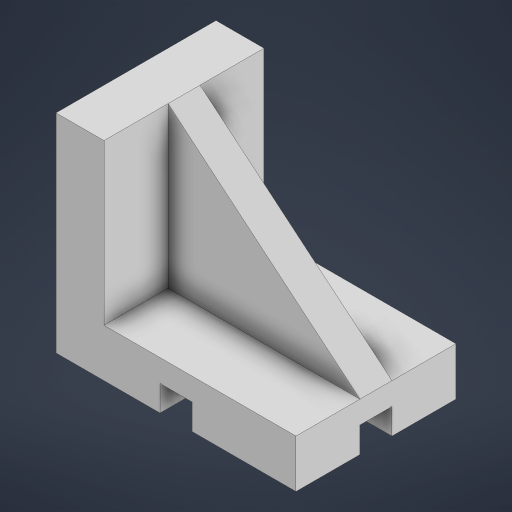
# Autodesk Inventor part: Part2
Saved by Autodesk Inventor 2023 (Build 270158000, 158)
## iProperties
Created: 2023-04-25
Part Number: Part2
Material: Ogólny
Document SubType Name: Modeling
Designer: Adam
Density: 1 g/cm^3
Appearance: Domyślna
Author: Adam
Autodesk Inventor part; units mm, degrees
ref_plane "YZ Plane" through (0, 0, 0) normal (1, 0, 0) x (0, 1, 0)
ref_plane "XZ Plane" through (0, 0, 0) normal (0, 1, 0) x (-1, 0, 0)
ref_plane "XY Plane" through (0, 0, 0) normal (0, 0, 1) x (1, 0, 0)
sketch "Szkic6" plane through (0, 0, 0) normal (0, 0, 1) x (1, 0, 0)
  point P0 (0, 0)
sketch "Szkic7" plane through (0, 0, 0) normal (0, 0, 1) x (1, 0, 0)
  line L0 (0, 65) -> (0, 0)
  line L1 (0, 0) -> (75, 0)
  line L2 (75, 0) -> (75, 15)
  line L3 (75, 15) -> (15, 15)
  line L4 (15, 15) -> (15, 65)
  line L5 (15, 65) -> (0, 65)
  dimension "d13" = 65
  dimension "d14" = 75
  dimension "d15" = 15
  dimension "d16" = 15
  constraints: 12 end point, 5 perpendicular, 1 vertical
  measures "d13" distance of L0.start L0.end
  measures "d14" distance of L0.end L1.end
  measures "d15" distance of L1.end L2.end
  measures "d16" distance of L4.end L0.start
extrude "Wyciągnięcie proste3" add sketch "Szkic7" along normal mid plane 50
sketch "Szkic8" plane through (0, 0, 0) normal (0, 0, 1) x (1, 0, 0)
  line L0 (15, 65) -> (0, 65) projected
  line L1 (75, 0) -> (75, 15) projected
  line L2 (15, 65) -> (75, 15)
  point P0 (0, 0)
  constraints: 2 end point
extrude "Żebro2" add sketch "Szkic8" along normal mid plane 10 rib yes fills toward (7.5, 64.95) open curves L0 L2 L1
sketch "Szkic9" plane through (0, 0, -25) normal (0, -1, 0) x (1, 0, 0)
  line L0 (0, 0) -> (0, 50) projected
  line L1 (15, 20) -> (75, 20) projected
  line L2 (0, 30) -> (75, 30)
  line L3 (75, 30) -> (75, 20)
  line L4 (75, 20) -> (0, 20)
  line L5 (0, 20) -> (0, 30)
  line L6 (75, 50) -> (15, 50) projected
  line L7 (15, 0) -> (75, 0) projected
  line L8 (32.5, 50) -> (42.5, 50)
  line L9 (42.5, 50) -> (42.5, 0)
  line L10 (42.5, 0) -> (32.5, 0)
  line L11 (32.5, 0) -> (32.5, 50)
  point P0 (0, 25)
  point P1 (32.5, 30)
  point P2 (0, 20)
  point P3 (32.5, 20)
  point P4 (32.5, 0)
  point P5 (42.5, 20)
  point P6 (42.5, 30)
  dimension "d25" = 10
  dimension "d26" = 10
  dimension "d27" = 32.5
  constraints: 16 end point, 4 parallel, 3 point on line, 2 horizontal, 2 perpendicular
  measures "d25" distance between parallel lines of L9 L11
  measures "d26" distance between parallel lines of L4 L2
  measures "d27" distance between parallel lines of L11 L0
extrude "Wyciągnięcie proste4" cut sketch "Szkic9" against normal blind 8
